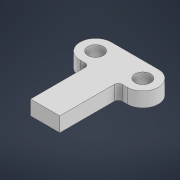
# Autodesk Inventor part: holder3_puller
Saved by Autodesk Inventor 2021 (Build 250183000, 183)
## iProperties
Created: 2021-06-13
Part Number: holder3_puller
Material: Generic
Document SubType Name: Modeling
Designer: Watchdog
Density: 1 g/cm^3
Appearance: Default
Author: Watchdog
Autodesk Inventor part; units mm, degrees
ref_plane "YZ Plane" through (0, 0, 0) normal (1, 0, 0) x (0, 1, 0)
ref_plane "XZ Plane" through (0, 0, 0) normal (0, 1, 0) x (-1, 0, 0)
ref_plane "XY Plane" through (0, 0, 0) normal (0, 0, 1) x (1, 0, 0)
sketch "Sketch1" plane through (0, 0, 0) normal (0, 1, 0) x (-1, 0, 0)
  line L0 (12.113, -8) -> (-12.113, -8)
  line L1 (-12.113, 8) -> (12.113, 8)
  arc A0 (12.113, -8) -> (12.113, 8) centre (12.113, 0) ccw
  arc A1 (-12.113, 8) -> (-12.113, -8) centre (-12.113, 0) ccw
  point P0 (0, 0)
  dimension "d0" = 16
  dimension "d2" = 8
  dimension "d4" = 24.226
  dimension "d5" = 12.113
  constraints: 4 end point, 4 point on circle, 4 tangent, 2 centre point, 1 horizontal
  measures "d0" distance between parallel lines of L1 L0
  measures "d2" distance from line of point (0, 0) L0
  measures "d4" distance of L0.end L0.start
  measures "d5" horizontal distance of point (0, 0) L0.start
extrude "Extrusion1" add sketch "Sketch1" along normal blind 7.5
sketch "Sketch2" plane through (0, 7.5, 0) normal (0, 1, 0) x (1, 0, 0)
  arc A0 (-12.113, 8) -> (-12.113, -8) centre (-12.113, 0) ccw projected
  arc A1 (12.113, -8) -> (12.113, 8) centre (12.113, 0) ccw projected
  point P0 (0, 0)
  point P1 (-12.113, 0)
  point P2 (12.113, 0)
  dimension "d8" = 0
  dimension "d9" = 0
  dimension "d11" = 0
  dimension "d12" = 0
  measures "d8" vertical distance of point (0, 0) point (-12.113, 0)
  measures "d9" vertical distance of point (0, 0) point (12.113, 0)
  measures "d11" distance of A0.centre point (-12.113, 0)
  measures "d12" distance of A1.centre point (12.113, 0)
hole "Hole1" at (12.113, 7.5, 0) at (-12.113, 7.5, 0) direction (0, -1, 0) diameter 8 end through all
sketch "Sketch3" plane through (-12.113, 0, 8) normal (0, 0, 1) x (1, 0, 0)
  line L0 (24.226, 7.5) -> (0, 7.5) projected
  line L1 (24.226, 0) -> (0, 0) projected
  line L2 (4.613, 7.5) -> (19.613, 7.5)
  line L3 (19.613, 7.5) -> (19.613, 0)
  line L4 (19.613, 0) -> (4.613, 0)
  line L5 (4.613, 0) -> (4.613, 7.5)
  point P0 (12.113, 0)
  point P1 (4.613, 0)
  dimension "d20" = 15
  dimension "d21" = 7.5
  constraints: 8 end point, 2 parallel, 2 point on line, 1 horizontal, 1 perpendicular
  measures "d20" distance between parallel lines of L3 L5
  measures "d21" distance from line of L5 point (12.113, 0)
extrude "Extrusion2" add sketch "Sketch3" along normal blind 30
fillet "Fillet1" radius 2 2 edges at (-7.5, 3.75, 8) (7.5, 3.75, 8)
equation "\"d2\" = 0.5 * d0"
equation "\"d5\" = 0.5 * d4"
equation "\"d21\" = 0.5 * d20"
body "Solid1"
